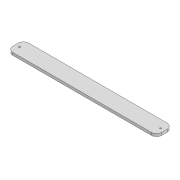
# Autodesk Inventor part: RWANDA_SIGN4
Saved by Autodesk Inventor 2021 (Build 250183000, 183)
## iProperties
Created: 2021-12-17
Part Number: RWANDA_SIGN4
Material: Generic
Document SubType Name: Modeling
Designer: Administrator
Density: 1 g/cm^3
Appearance: Default
Author: Administrator
Autodesk Inventor part; units mm, degrees
ref_plane "YZ Plane" through (0, 0, 0) normal (1, 0, 0) x (0, 1, 0)
ref_plane "XZ Plane" through (0, 0, 0) normal (0, 1, 0) x (-1, 0, 0)
ref_plane "XY Plane" through (0, 0, 0) normal (0, 0, 1) x (1, 0, 0)
sketch "Sketch1" plane through (0, 0, 0) normal (0, 1, 0) x (-1, 0, 0)
  line L0 (-243.1605, 15) -> (243.1604, 15) construction
  line L1 (243.1604, 15) -> (243.1604, -15) construction
  line L2 (243.1604, -15) -> (-243.1605, -15) construction
  line L3 (-243.1605, -15) -> (-243.1605, 15) construction
  line L4 (-214.4004, -15) -> (-218.3874, -15)
  line L5 (-218.3874, -15) -> (-218.3874, 10.8428)
  line L6 (-218.3874, 10.8428) -> (-226.2156, -6.7342)
  line L7 (-226.2156, -6.7342) -> (-228.6467, -6.7342)
  line L8 (-228.6467, -6.7342) -> (-236.402, 10.8428)
  line L9 (-236.402, 10.8428) -> (-236.402, -15)
  line L10 (-236.402, -15) -> (-240.1216, -15)
  line L11 (-240.1216, -15) -> (-240.1216, 15)
  line L12 (-240.1216, 15) -> (-234.6759, 15)
  line L13 (-234.6759, 15) -> (-227.1881, -1.7018)
  line L14 (-227.1881, -1.7018) -> (-219.9433, 15)
  line L15 (-219.9433, 15) -> (-214.4004, 15)
  line L16 (-214.4004, 15) -> (-214.4004, -15)
  line L17 (-198.671, -15) -> (-188.5576, 15)
  line L18 (-188.5576, 15) -> (-183.6467, 15)
  line L19 (-183.6467, 15) -> (-173.5333, -15)
  line L20 (-173.5333, -15) -> (-177.7391, -15)
  line L21 (-177.7391, -15) -> (-180.462, -6.6126)
  line L22 (-180.462, -6.6126) -> (-191.9125, -6.6126)
  line L23 (-191.9125, -6.6126) -> (-194.6354, -15)
  line L24 (-194.6354, -15) -> (-198.671, -15)
  line L25 (-181.556, -3.2091) -> (-186.1994, 10.9157)
  line L26 (-186.1994, 10.9157) -> (-190.8185, -3.2091)
  line L27 (-190.8185, -3.2091) -> (-181.556, -3.2091)
  spline S0 degree 2 poles (-134.1492, -0.0243) (-134.1492, -4.1329) (-137.4798, -10.7455) (-140.2756, -12.5932) knots 0 0 0 1 2 2 2
  spline S1 degree 2 poles (-140.2756, -12.5932) (-142.5608, -14.0276) (-147.2529, -15) (-150.8996, -15) knots 0 0 0 1 2 2 2
  line L28 (-150.8996, -15) -> (-157.8039, -15)
  line L29 (-157.8039, -15) -> (-157.8039, 15)
  line L30 (-157.8039, 15) -> (-150.9725, 15)
  spline S2 degree 2 poles (-150.9725, 15) (-146.7423, 15) (-141.9287, 13.7358) (-140.227, 12.6175) knots 0 0 0 1 2 2 2
  spline S3 degree 2 poles (-140.227, 12.6175) (-137.3339, 10.6969) (-134.1492, 4.3517) (-134.1492, -0.0243) knots 0 0 0 1 2 2 2
  spline S4 degree 2 poles (-138.3064, 0.0243) (-138.3064, 3.4765) (-140.5916, 8.363) (-142.8526, 9.7488) knots 0 0 0 1 2 2 2
  spline S5 degree 2 poles (-142.8526, 9.7488) (-144.4571, 10.6969) (-148.0795, 11.5478) (-150.778, 11.5478) knots 0 0 0 1 2 2 2
  line L31 (-150.778, 11.5478) -> (-153.8169, 11.5478)
  line L32 (-153.8169, 11.5478) -> (-153.8169, -11.5478)
  line L33 (-153.8169, -11.5478) -> (-150.778, -11.5478)
  spline S6 degree 2 poles (-150.778, -11.5478) (-148.1281, -11.5478) (-144.1167, -10.6969) (-142.4879, -9.5543) knots 0 0 0 1 2 2 2
  spline S7 degree 2 poles (-142.4879, -9.5543) (-140.3971, -8.1442) (-138.3064, -3.4765) (-138.3064, 0.0243) knots 0 0 0 1 2 2 2
  line L34 (-116.9368, -15) -> (-116.9368, 15)
  line L35 (-116.9368, 15) -> (-98.1686, 15)
  line L36 (-98.1686, 15) -> (-98.1686, 11.4506)
  line L37 (-98.1686, 11.4506) -> (-112.9498, 11.4506)
  line L38 (-112.9498, 11.4506) -> (-112.9498, 3.2334)
  line L39 (-112.9498, 3.2334) -> (-99.1654, 3.2334)
  line L40 (-99.1654, 3.2334) -> (-99.1654, -0.316)
  line L41 (-99.1654, -0.316) -> (-112.9498, -0.316)
  line L42 (-112.9498, -0.316) -> (-112.9498, -11.4506)
  line L43 (-112.9498, -11.4506) -> (-98.1686, -11.4506)
  line L44 (-98.1686, -11.4506) -> (-98.1686, -15)
  line L45 (-98.1686, -15) -> (-116.9368, -15)
  line L46 (-57.5689, -15) -> (-69.1897, -15)
  line L47 (-69.1897, -15) -> (-69.1897, -11.9368)
  line L48 (-69.1897, -11.9368) -> (-65.3728, -11.9368)
  line L49 (-65.3728, -11.9368) -> (-65.3728, 11.9368)
  line L50 (-65.3728, 11.9368) -> (-69.1897, 11.9368)
  line L51 (-69.1897, 11.9368) -> (-69.1897, 15)
  line L52 (-69.1897, 15) -> (-57.5689, 15)
  line L53 (-57.5689, 15) -> (-57.5689, 11.9368)
  line L54 (-57.5689, 11.9368) -> (-61.3858, 11.9368)
  line L55 (-61.3858, 11.9368) -> (-61.3858, -11.9368)
  line L56 (-61.3858, -11.9368) -> (-57.5689, -11.9368)
  line L57 (-57.5689, -11.9368) -> (-57.5689, -15)
  line L58 (-18.2821, -15) -> (-22.7553, -15)
  line L59 (-22.7553, -15) -> (-36.0292, 10.8671)
  line L60 (-36.0292, 10.8671) -> (-36.0292, -15)
  line L61 (-36.0292, -15) -> (-39.7488, -15)
  line L62 (-39.7488, -15) -> (-39.7488, 15)
  line L63 (-39.7488, 15) -> (-34.0843, 15)
  line L64 (-34.0843, 15) -> (-22.0017, -8.752)
  line L65 (-22.0017, -8.752) -> (-22.0017, 15)
  line L66 (-22.0017, 15) -> (-18.2821, 15)
  line L67 (-18.2821, 15) -> (-18.2821, -15)
  line L68 (36.7828, -15) -> (31.6045, -15)
  line L69 (31.6045, -15) -> (22.1231, -3.0632)
  line L70 (22.1231, -3.0632) -> (17.5526, -3.0632)
  line L71 (17.5526, -3.0632) -> (17.5526, -15)
  line L72 (17.5526, -15) -> (13.5656, -15)
  line L73 (13.5656, -15) -> (13.5656, 15)
  line L74 (13.5656, 15) -> (21.2966, 15)
  spline S8 degree 2 poles (21.2966, 15) (23.8735, 15) (27.35, 14.4408) (28.9303, 13.4198) knots 0 0 0 1 2 2 2
  spline S9 degree 2 poles (28.9303, 13.4198) (30.5105, 12.3987) (32.3338, 9.2139) (32.3338, 6.8558) knots 0 0 0 1 2 2 2
  spline S10 degree 2 poles (32.3338, 6.8558) (32.3338, 3.5737) (28.9789, -0.8752) (26.1102, -1.9449) knots 0 0 0 1 2 2 2
  line L75 (26.1102, -1.9449) -> (36.7828, -15)
  spline S11 degree 2 poles (28.1766, 6.5397) (28.1766, 7.8525) (27.2528, 9.8703) (26.2803, 10.5267) knots 0 0 0 1 2 2 2
  spline S12 degree 2 poles (26.2803, 10.5267) (25.4295, 11.0859) (23.1685, 11.5478) (21.5154, 11.5478) knots 0 0 0 1 2 2 2
  line L76 (21.5154, 11.5478) -> (17.5526, 11.5478)
  line L77 (17.5526, 11.5478) -> (17.5526, 0.2674)
  line L78 (17.5526, 0.2674) -> (21.0534, 0.2674)
  spline S13 degree 2 poles (21.0534, 0.2674) (22.7795, 0.2674) (25.5267, 0.8752) (26.4748, 1.8233) knots 0 0 0 1 2 2 2
  spline S14 degree 2 poles (26.4748, 1.8233) (27.35, 2.6499) (28.1766, 4.9838) (28.1766, 6.5397) knots 0 0 0 1 2 2 2
  line L79 (85.6726, 15) -> (78.1361, -15)
  line L80 (78.1361, -15) -> (73.6628, -15)
  line L81 (73.6628, -15) -> (67.5607, 9.8947)
  line L82 (67.5607, 9.8947) -> (61.6288, -15)
  line L83 (61.6288, -15) -> (57.2042, -15)
  line L84 (57.2042, -15) -> (49.5461, 15)
  line L85 (49.5461, 15) -> (53.6547, 15)
  line L86 (53.6547, 15) -> (59.6839, -9.8703)
  line L87 (59.6839, -9.8703) -> (65.6645, 15)
  line L88 (65.6645, 15) -> (69.7244, 15)
  line L89 (69.7244, 15) -> (75.7536, -10.1621)
  line L90 (75.7536, -10.1621) -> (81.7585, 15)
  line L91 (81.7585, 15) -> (85.6726, 15)
  line L92 (98.8978, -15) -> (109.0113, 15)
  line L93 (109.0113, 15) -> (113.9222, 15)
  line L94 (113.9222, 15) -> (124.0356, -15)
  line L95 (124.0356, -15) -> (119.8298, -15)
  line L96 (119.8298, -15) -> (117.1069, -6.6126)
  line L97 (117.1069, -6.6126) -> (105.6564, -6.6126)
  line L98 (105.6564, -6.6126) -> (102.9335, -15)
  line L99 (102.9335, -15) -> (98.8978, -15)
  line L100 (116.0129, -3.2091) -> (111.3695, 10.9157)
  line L101 (111.3695, 10.9157) -> (106.7504, -3.2091)
  line L102 (106.7504, -3.2091) -> (116.0129, -3.2091)
  line L103 (161.2317, -15) -> (156.7585, -15)
  line L104 (156.7585, -15) -> (143.4846, 10.8671)
  line L105 (143.4846, 10.8671) -> (143.4846, -15)
  line L106 (143.4846, -15) -> (139.7649, -15)
  line L107 (139.7649, -15) -> (139.7649, 15)
  line L108 (139.7649, 15) -> (145.4295, 15)
  line L109 (145.4295, 15) -> (157.5121, -8.752)
  line L110 (157.5121, -8.752) -> (157.5121, 15)
  line L111 (157.5121, 15) -> (161.2317, 15)
  line L112 (161.2317, 15) -> (161.2317, -15)
  spline S15 degree 2 poles (203.8492, -0.0243) (203.8492, -4.1329) (200.5186, -10.7455) (197.7228, -12.5932) knots 0 0 0 1 2 2 2
  spline S16 degree 2 poles (197.7228, -12.5932) (195.4376, -14.0276) (190.7455, -15) (187.0988, -15) knots 0 0 0 1 2 2 2
  line L113 (187.0988, -15) -> (180.1944, -15)
  line L114 (180.1944, -15) -> (180.1944, 15)
  line L115 (180.1944, 15) -> (187.0259, 15)
  spline S17 degree 2 poles (187.0259, 15) (191.256, 15) (196.0696, 13.7358) (197.7714, 12.6175) knots 0 0 0 1 2 2 2
  spline S18 degree 2 poles (197.7714, 12.6175) (200.6645, 10.6969) (203.8492, 4.3517) (203.8492, -0.0243) knots 0 0 0 1 2 2 2
  spline S19 degree 2 poles (199.692, 0.0243) (199.692, 3.4765) (197.4068, 8.363) (195.1458, 9.7488) knots 0 0 0 1 2 2 2
  spline S20 degree 2 poles (195.1458, 9.7488) (193.5413, 10.6969) (189.9189, 11.5478) (187.2204, 11.5478) knots 0 0 0 1 2 2 2
  line L116 (187.2204, 11.5478) -> (184.1815, 11.5478)
  line L117 (184.1815, 11.5478) -> (184.1815, -11.5478)
  line L118 (184.1815, -11.5478) -> (187.2204, -11.5478)
  spline S21 degree 2 poles (187.2204, -11.5478) (189.8703, -11.5478) (193.8816, -10.6969) (195.5105, -9.5543) knots 0 0 0 1 2 2 2
  spline S22 degree 2 poles (195.5105, -9.5543) (197.6013, -8.1442) (199.692, -3.4765) (199.692, 0.0243) knots 0 0 0 1 2 2 2
  line L119 (217.8282, -15) -> (227.9416, 15)
  line L120 (227.9416, 15) -> (232.8525, 15)
  line L121 (232.8525, 15) -> (242.9659, -15)
  line L122 (242.9659, -15) -> (238.7601, -15)
  line L123 (238.7601, -15) -> (236.0372, -6.6126)
  line L124 (236.0372, -6.6126) -> (224.5867, -6.6126)
  line L125 (224.5867, -6.6126) -> (221.8638, -15)
  line L126 (221.8638, -15) -> (217.8282, -15)
  line L127 (234.9432, -3.2091) -> (230.2998, 10.9157)
  line L128 (230.2998, 10.9157) -> (225.6807, -3.2091)
  line L129 (225.6807, -3.2091) -> (234.9432, -3.2091)
  point P0 (0, 0)
  dimension "d3" = 15
  dimension "d4" = 243.1605
  constraints: 2 other
  measures "d3" distance from line of point (0, 0) L0
  measures "d4" distance from line of point (0, 0) L3
extrude "Extrusion1" add sketch "Sketch1" against normal blind 5
sketch "Sketch2" plane through (0, 0, 0) normal (0, 1, 0) x (1, 0, 0)
  line L0 (280, 30) -> (-280, 30)
  line L1 (-280, 30) -> (-280, -30)
  line L2 (-280, -30) -> (280, -30)
  line L3 (280, -30) -> (280, 30)
  line L4 (280, 30) -> (-280, -30) construction
  line L5 (-280, 30) -> (280, -30) construction
  point P0 (0, 0)
  dimension "d7" = 560
  dimension "d8" = 60
  constraints: 12 end point, 2 midpoint, 2 parallel, 1 horizontal, 1 perpendicular
  measures "d7" distance of L2.end L1.end
  measures "d8" distance of L1.end L0.end
extrude "Extrusion2" add sketch "Sketch2" along normal blind 10
fillet "Fillet1" radius 20 4 edges at (280, 5, -30) (280, 5, 30) (-280, 5, 30) (-280, 5, -30)
sketch "Sketch3" plane through (0, 0, 0) normal (0, -1, 0) x (1, 0, 0)
  line L0 (-280, -10) -> (-280, 10) projected
  line L1 (280, 10) -> (280, -10) projected
  point P0 (0, 0)
  point P1 (-265, 0)
  point P2 (265, 0)
  dimension "d12" = 15
  dimension "d13" = 15
  measures "d12" distance from line of L0 point (-265, 0)
  measures "d13" distance from line of L1 point (265, 0)
hole "Hole1" at (-265, 0, 0) at (265, 0, 0) direction (0, 1, 0) diameter 5.5 end through all countersink diameter 10.4 countersink angle 90 clearance for "Countersunk Flat Head Screw ISO 2009/7046" size "M5" standard "ISO"
body "Solid1"
